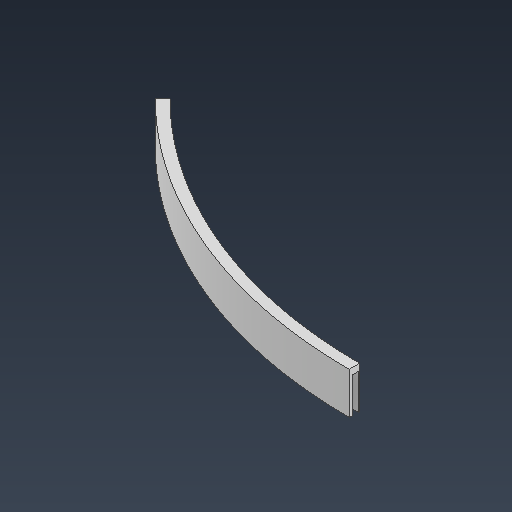
# Autodesk Inventor part: 23
Saved by Autodesk Inventor 2026 (Build 300175000, 175)
## iProperties
Created: 2026-09-23
Part Number: 23
Material: 一般
Document SubType Name: Modeling
Designer: nozomi
Density: 1 g/cm^3
Appearance: 既定
Author: nozomi
Autodesk Inventor part; units mm, degrees
ref_plane "YZ Plane" through (0, 0, 0) normal (1, 0, 0) x (0, 1, 0)
ref_plane "XZ Plane" through (0, 0, 0) normal (0, 1, 0) x (-1, 0, 0)
ref_plane "XY Plane" through (0, 0, 0) normal (0, 0, 1) x (1, 0, 0)
sketch "スケッチ1" plane through (0, 0, 0) normal (0, 1, 0) x (-1, 0, 0)
  circle A0 centre (0, 0) radius 287.828
  circle A1 centre (0, 0) radius 289.328
  line L0 (204.5858, 204.5858) -> (0, 0)
  line L1 (0, 0) -> (0, 289.328)
  point P0 (0, 287.828)
  point P1 (203.5251, 203.5251)
  dimension "d0" = 575.656
  dimension "d1" = 578.656
  dimension "d2" = 45
  constraints: 4 end point, 2 centre point, 2 coincident, 2 point on circle, 1 vertical alignment
  measures "d0" diameter of A0
  measures "d1" diameter of A1
  measures "d2" angle of L1 L0
extrude "押し出し1" add sketch "スケッチ1" along normal blind 14 contours A0 L1 A1 L0 picked at (198.6715, 209.3726)
sketch "スケッチ2" plane through (0, 14, 0) normal (0, 1, 0) x (1, 0, 0)
  arc A0 (-203.5251, -203.5251) -> (0, -287.828) centre (0, 0) ccw projected
  line L0 (-203.5251, -203.5251) -> (-204.5858, -204.5858) projected
  arc A1 (-204.5858, -204.5858) -> (0, -289.328) centre (0, 0) ccw projected
  line L1 (0, -289.328) -> (0, -287.828) projected
  circle A2 centre (0, 0) radius 286.828
  circle A3 centre (0, 0) radius 285.828
  circle A4 centre (0, 0) radius 290.328
  circle A5 centre (0, 0) radius 292.328
  line L2 (-206.7071, -206.7071) -> (-202.1109, -202.1109)
  line L3 (0, -292.328) -> (0, -285.828)
  point P0 (0, -290.328)
  point P1 (-205.2929, -205.2929)
  point P2 (0, -286.828)
  point P3 (-202.818, -202.818)
  dimension "d5" = 1
  dimension "d6" = 1
  dimension "d7" = 1
  dimension "d8" = 2
  constraints: 4 centre point, 4 coincident, 4 end point, 4 point on circle, 2 collinear, 1 vertical
  measures "d5" radial gap between concentric circles of A2 A0
  measures "d6" radial gap between concentric circles of A2 A3
  measures "d7" radial gap between concentric circles of A4 A1
  measures "d8" radial gap between concentric circles of A5 A4
extrude "押し出し2" add sketch "スケッチ2" against normal up to surface (14 mm away) contours L2 A3 L3 A2 | A4 L3 A5 L2 picked at (-162.1553, -235.9498) picked at (-183.4103, -226.5178)
sketch "スケッチ3" plane through (0, 14, 0) normal (0, 1, 0) x (1, 0, 0)
  arc A0 (-205.2929, -205.2929) -> (0, -290.328) centre (0, 0) ccw projected
  line L0 (-205.2929, -205.2929) -> (-206.7071, -206.7071) projected
  arc A1 (-206.7071, -206.7071) -> (0, -292.328) centre (0, 0) ccw projected
  line L1 (0, -292.328) -> (0, -290.328) projected
  arc A2 (-203.5251, -203.5251) -> (0, -287.828) centre (0, 0) ccw projected
  arc A3 (-203.5251, -203.5251) -> (0, -287.828) centre (0, 0) ccw projected
  line L2 (-203.5251, -203.5251) -> (-204.5858, -204.5858) projected
  arc A4 (-204.5858, -204.5858) -> (0, -289.328) centre (0, 0) ccw projected
  line L3 (0, -289.328) -> (0, -287.828) projected
  arc A5 (-202.1109, -202.1109) -> (0, -285.828) centre (0, 0) ccw projected
  line L4 (-202.1109, -202.1109) -> (-202.818, -202.818) projected
  arc A6 (-202.818, -202.818) -> (0, -286.828) centre (0, 0) ccw projected
  line L5 (0, -286.828) -> (0, -285.828) projected
  line L6 (-206.7071, -206.7071) -> (-202.1109, -202.1109)
  line L7 (0, -286.828) -> (0, -292.328)
  constraints: 4 end point, 1 vertical
extrude "押し出し3" add sketch "スケッチ3" along normal blind 12
extrude "押し出し4" cut sketch "スケッチ1" along normal up to surface (14 mm away) contours A0 L1 A1 L0 picked at (198.6715, 209.3726)
sketch "スケッチ4" plane through (0, 14, 0) normal (0, -1, 0) x (1, 0, 0)
  line L0 (-202.818, 202.818) -> (-205.2929, 205.2929) projected
  arc A0 (0, 286.828) -> (-202.818, 202.818) centre (0, 0) ccw projected
  line L1 (0, 290.328) -> (0, 286.828) projected
  arc A1 (0, 290.328) -> (-205.2929, 205.2929) centre (0, 0) ccw projected
extrude "押し出し5" cut sketch "スケッチ4" against normal blind 8
equation "\"d7\" = d5"
